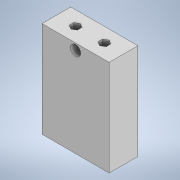
# Autodesk Inventor part: bumper piece 1
Saved by Autodesk Inventor 2022 (Build 260153000, 153)
## iProperties
Created: 2023-01-09
Part Number: bumper piece 1
Material: Generic
Document SubType Name: Modeling
Designer: s143573
Density: 1 g/cm^3
Appearance: Default
Author: s143573
Autodesk Inventor part; units mm, degrees
ref_plane "YZ Plane" through (0, 0, 0) normal (1, 0, 0) x (0, 1, 0)
ref_plane "XZ Plane" through (0, 0, 0) normal (0, 1, 0) x (-1, 0, 0)
ref_plane "XY Plane" through (0, 0, 0) normal (0, 0, 1) x (1, 0, 0)
sketch "Sketch2" plane through (0, 0, 0) normal (0, 1, 0) x (-1, 0, 0)
  line L0 (0, 0) -> (44.45, 0)
  line L1 (44.45, 0) -> (44.45, -19.05)
  line L2 (44.45, -19.05) -> (0, -19.05)
  line L3 (0, -19.05) -> (0, 0)
  dimension "d2" = 19.05
  dimension "d3" = 44.45
  constraints: 8 end point, 2 parallel, 1 horizontal, 1 perpendicular
  measures "d2" distance of L0.end L1.end
  measures "d3" distance of L1.end L2.end
extrude "Extrusion2" add sketch "Sketch2" along normal blind 63.5
sketch "Sketch6" plane through (0, 63.5, 0) normal (0, 1, 0) x (1, 0, 0)
  line L0 (-44.45, 19.05) -> (-44.45, 0) projected
  line L1 (-44.45, 9.525) -> (0, 9.525)
  line L2 (0, 0) -> (0, 19.05) projected
  line L3 (-31.8, 12.7) -> (-29.0254, 11.1558)
  line L4 (-29.0254, 11.1558) -> (-28.9754, 7.9808)
  line L5 (-28.9754, 7.9808) -> (-31.7, 6.35)
  line L6 (-31.7, 6.35) -> (-34.4746, 7.8942)
  line L7 (-34.4746, 7.8942) -> (-34.5246, 11.0692)
  line L8 (-34.5246, 11.0692) -> (-31.8, 12.7)
  line L9 (-15.5043, 11.0178) -> (-12.8093, 12.7)
  line L10 (-12.8093, 12.7) -> (-10.005, 11.2072)
  line L11 (-10.005, 11.2072) -> (-9.8957, 8.0322)
  line L12 (-9.8957, 8.0322) -> (-12.5907, 6.35)
  line L13 (-12.5907, 6.35) -> (-15.395, 7.8428)
  line L14 (-15.395, 7.8428) -> (-15.5043, 11.0178)
  point P0 (-31.75, 9.525)
  point P1 (-12.7, 9.525)
  dimension "d17" = 44.45
  dimension "d18" = 6.35
  dimension "d19" = 6.35
  dimension "d20" = 12.7
  dimension "d21" = 12.7
  constraints: 26 end point, 2 midpoint, 2 point on line, 26 other
  measures "d17" distance of L1.start L1.end
  measures "d18" vertical distance of L3.start L5.end
  measures "d19" vertical distance of L9.end L12.end
  measures "d20" distance of L1.start point (-31.75, 9.525)
  measures "d21" distance of L1.end point (-12.7, 9.525)
extrude "Extrusion3" cut sketch "Sketch6" against normal blind 50.8
sketch "Sketch15" plane through (-44.45, 0, 0) normal (0, 0, 1) x (1, 0, 0)
  circle A0 centre (22.225, 59.2325) radius 3.3782
  line L0 (0, 0) -> (0, 63.5) projected
  point P0 (44.45, 0)
  dimension "d49" = 22.225
  dimension "d50" = 6.7564
  constraints: 1 centre point
  measures "d49" distance from line of A0.centre L0
  measures "d50" diameter of A0
extrude "Extrusion9" cut sketch "Sketch15" against normal blind 25.4
body "Solid2"
